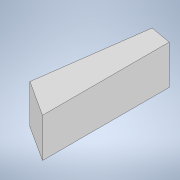
# Autodesk Inventor part: FP Side Boards
Saved by Autodesk Inventor 2020 (Build 240168000, 168)
## iProperties
Created: 2021-04-23
Part Number: FP Side Boards
Material: Generic
Document SubType Name: Modeling
Designer: austi
Density: 1 g/cm^3
Appearance: Default
Author: austi
Autodesk Inventor part; units mm, degrees
ref_plane "YZ Plane" through (0, 0, 0) normal (1, 0, 0) x (0, 1, 0)
ref_plane "XZ Plane" through (0, 0, 0) normal (0, 1, 0) x (-1, 0, 0)
ref_plane "XY Plane" through (0, 0, 0) normal (0, 0, 1) x (1, 0, 0)
sketch "Sketch1" plane through (0, 0, 0) normal (0, 1, 0) x (-1, 0, 0)
  line L0 (0, 0) -> (0, -42)
  line L1 (0, -42) -> (6.8875, -43.25)
  line L2 (6.8875, -43.25) -> (11.7689, -7.5825)
  line L3 (11.7689, -7.5825) -> (0, 0)
  line L4 (14.1226, 0) -> (-2.3538, 0) projected
  line L5 (0, -51.9) -> (0, 8.65) projected
  dimension "d0" = 42
  dimension "d1" = 7
  dimension "d2" = 36
  dimension "d3" = 14
  dimension "d4" = 115
  dimension "d5" = 79.713
  constraints: 8 end point, 1 vertical
  measures "d0" distance of L0.start L0.end
  measures "d1" distance of L0.end L1.end
  measures "d2" distance of L1.end L2.end
  measures "d3" distance of L0.start L2.end
  measures "d4" angle of L3 L2
  measures "d5" angle of L5 L1
extrude "Extrusion1" add sketch "Sketch1" along normal blind 13
body "Solid1"
